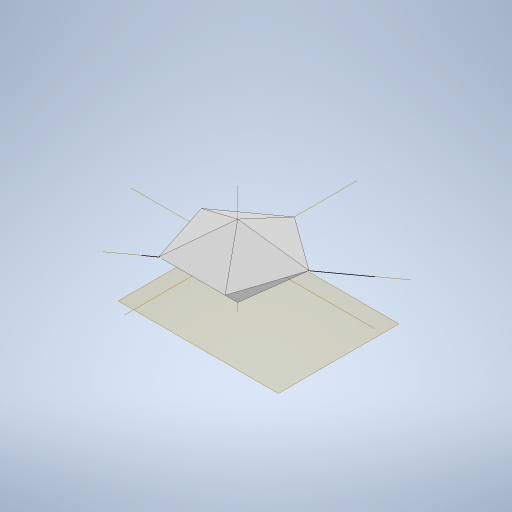
# Autodesk Inventor part: D20-2
Saved by Autodesk Inventor 2023 (Build 270158030, 158C)
## iProperties
Created: 2024-08-24
Part Number: D20-2
Material: Generic
Document SubType Name: Modeling
Designer: Imogen Heard
Density: 1 g/cm^3
Appearance: Default
Author: Imogen Heard
Autodesk Inventor part; units mm, degrees
ref_plane "YZ Plane" through (0, 0, 0) normal (1, 0, 0) x (0, 1, 0)
ref_plane "XY Plane" through (0, 0, 0) normal (0, 0, 1) x (1, 0, 0)
sketch "Sketch3" plane through (0, 0, 0) normal (0, 1, 0) x (-1, 0, 0)
  line L0 (-12.9968, 17.8885) -> (12.9968, 17.8885)
  line L1 (12.9968, 17.8885) -> (21.0292, -6.8328)
  line L2 (21.0292, -6.8328) -> (0, -22.1115)
  line L3 (0, -22.1115) -> (-21.0292, -6.8328)
  line L4 (-21.0292, -6.8328) -> (-12.9968, 17.8885)
  point P0 (0, 0)
  point P1 (0, 0)
  dimension "d15" = 40
  constraints: 10 end point, 1 coincident, 1 horizontal, 11 other
  measures "d15" distance from line of L2.end L0
extrude "Extrusion2" add sketch "Sketch3" along normal blind 20 draft -60
sketch "Sketch4" plane through (0, 0, 0) normal (0, 1, 0) x (-1, 0, 0)
  line L0 (16.8704, 20.7029) -> (-35.8904, -17.6301)
  point P0 (0, 0)
  point P1 (-21.0292, -6.8328)
  point P2 (12.9968, 17.8885)
  constraints: 2 end point, 2 point on line
sketch "Sketch5" plane through (0, 0, 0) normal (0, -1, 0) x (1, 0, 0)
  line L0 (21.0292, -6.8328) -> (0, -22.1115) projected
  line L1 (12.9968, 17.8885) -> (21.0292, -6.8328) projected
  line L2 (-12.9968, 17.8885) -> (12.9968, 17.8885) projected
  line L3 (-21.0292, -6.8328) -> (-12.9968, 17.8885) projected
  line L4 (0, -22.1115) -> (-21.0292, -6.8328) projected
  point P0 (0, 0)
extrude "Extrusion3" add sketch "Sketch5" along normal blind 20 draft -45
ref_plane "Work Plane3" through (0, -17.8885, 0) normal (0, 1, 0) x (-1, 0, 0)
body "Solid2"
